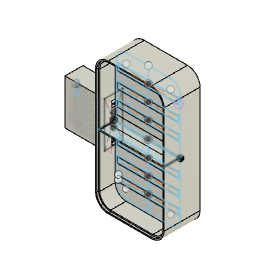
Sign (Autodesk Fusion 360 design; units mm, degrees)
Autodesk Fusion 360 part; units mm, degrees
note: some values were not read from the file. Chosen so that the rebuilt part matches the saved one: which face or edge a step refers to. Set by a fixed rule: which sketch regions a step uses.
sketch "body" plane through (0, 0, 0) normal (0, 1, 0) x (1, 0, 0)
  line L0 (36, 110) -> (-36, 110)
  line L1 (-57, 89) -> (-57, -89)
  line L2 (-36, -110) -> (36, -110)
  line L3 (57, -89) -> (57, 89)
  line L4 (57, 110) -> (-57, -110) construction
  line L5 (-57, 110) -> (57, -110) construction
  arc A0 (-57, -89) -> (-36, -110) centre (-36, -89) ccw
  arc A1 (36, -110) -> (57, -89) centre (36, -89) ccw
  arc A2 (57, 89) -> (36, 110) centre (36, 89) ccw
  arc A3 (-36, 110) -> (-57, 89) centre (-36, 89) ccw
  line L6 (-35.2, -106.2) -> (35.2, -106.2)
  line L7 (53.2, -88.2) -> (53.2, 88.2)
  line L8 (35.2, 106.2) -> (-35.2, 106.2)
  line L9 (-53.2, 88.2) -> (-53.2, -88.2)
  line L10 (-53.2, -106.2) -> (53.2, 106.2) construction
  line L11 (53.2, -106.2) -> (-53.2, 106.2) construction
  arc A4 (-53.2, -88.2) -> (-35.2, -106.2) centre (-35.2, -88.2) ccw
  arc A5 (35.2, -106.2) -> (53.2, -88.2) centre (35.2, -88.2) ccw
  arc A6 (-35.2, 106.2) -> (-53.2, 88.2) centre (-35.2, 88.2) ccw
  arc A7 (53.2, 88.2) -> (35.2, 106.2) centre (35.2, 88.2) ccw
  line L12 (35.2, 108.2) -> (-35.2, 108.2)
  line L13 (-55.2, 88.2) -> (-55.2, -88.2)
  line L14 (-35.2, -108.2) -> (35.2, -108.2)
  line L15 (55.2, -88.2) -> (55.2, 88.2)
  line L16 (55.2, 108.2) -> (-55.2, -108.2) construction
  line L17 (-55.2, 108.2) -> (55.2, -108.2) construction
  arc A8 (-55.2, -88.2) -> (-35.2, -108.2) centre (-35.2, -88.2) ccw
  arc A9 (35.2, -108.2) -> (55.2, -88.2) centre (35.2, -88.2) ccw
  arc A10 (55.2, 88.2) -> (35.2, 108.2) centre (35.2, 88.2) ccw
  arc A11 (-35.2, 108.2) -> (-55.2, 88.2) centre (-35.2, 88.2) ccw
  line L18 (-55, -1) -> (55, -1)
  line L19 (55, -1) -> (55, 1)
  line L20 (55, 1) -> (-55, 1)
  line L21 (-55, 1) -> (-55, -1)
  line L22 (-55, -1) -> (55, 1) construction
  line L23 (55, -1) -> (-55, 1) construction
  dimension "d1" = 220
  dimension "d2" = 114
  dimension "d3" = 21
  dimension "d4" = 21
  dimension "d5" = 21
  dimension "d6" = 21
  dimension "d10" = 106.4
  dimension "d11" = 212.4
  dimension "d12" = 18
  dimension "d13" = 18
  dimension "d14" = 18
  dimension "d15" = 18
  dimension "d48" = 110.4
  dimension "d49" = 216.4
  dimension "d50" = 20
  dimension "d51" = 20
  dimension "d52" = 20
  dimension "d53" = 20
  dimension "d65" = 2
  dimension "d76" = 110
  constraint perpendicular L0 L1
  constraint parallel L0 L2
  constraint parallel L1 L3
  constraint horizontal L0
  constraint coincident L4 origin
  constraint coincident L5 origin
  constraint coincident L4.end L2
  constraint coincident L4.end L1
  constraint tangent L2 A0
  constraint tangent L1 A0
  constraint coincident L5.end L2
  constraint coincident L5.end L3
  constraint tangent L2 A1
  constraint tangent L3 A1
  constraint coincident L4.start L3
  constraint coincident L4.start L0
  constraint tangent L3 A2
  constraint tangent L0 A2
  constraint coincident L5.start L1
  constraint coincident L5.start L0
  constraint tangent L1 A3
  constraint tangent L0 A3
  constraint perpendicular L6 L7
  constraint parallel L6 L8
  constraint parallel L7 L9
  constraint horizontal L6
  constraint coincident L10 origin
  constraint coincident L11 origin
  constraint coincident L10.start L6
  constraint coincident L10.start L9
  constraint tangent L6 A4
  constraint tangent L9 A4
  constraint coincident L11.start L6
  constraint coincident L11.start L7
  constraint tangent L6 A5
  constraint tangent L7 A5
  constraint coincident L11.end L9
  constraint coincident L11.end L8
  constraint tangent L9 A6
  constraint tangent L8 A6
  constraint coincident L10.end L7
  constraint coincident L10.end L8
  constraint tangent L7 A7
  constraint tangent L8 A7
  constraint perpendicular L12 L13
  constraint parallel L12 L14
  constraint parallel L13 L15
  constraint horizontal L12
  constraint coincident L16 origin
  constraint coincident L17 origin
  constraint coincident L16.end L14
  constraint coincident L16.end L13
  constraint tangent L14 A8
  constraint tangent L13 A8
  constraint coincident L17.end L14
  constraint coincident L17.end L15
  constraint tangent L14 A9
  constraint tangent L15 A9
  constraint coincident L16.start L12
  constraint coincident L16.start L15
  constraint tangent L12 A10
  constraint tangent L15 A10
  constraint coincident L17.start L13
  constraint coincident L17.start L12
  constraint tangent L13 A11
  constraint tangent L12 A11
  constraint perpendicular L18 L19
  constraint parallel L18 L20
  constraint parallel L19 L21
  constraint horizontal L18
  constraint coincident L22 origin
  constraint coincident L23 origin
  measures "d1" distance of L5.start L4.end
  measures "d2" distance of L4.end L5.end
  measures "d3" radius of A0
  measures "d4" radius of A1
  measures "d5" radius of A2
  measures "d6" radius of A3
  measures "d10" distance of L10.end L11.end
  measures "d11" distance of L11.start L10.end
  measures "d12" radius of A4
  measures "d13" radius of A5
  measures "d14" radius of A6
  measures "d15" radius of A7
  measures "d48" distance of L16.end L17.end
  measures "d49" distance of L17.start L16.end
  measures "d50" radius of A8
  measures "d51" radius of A9
  measures "d52" radius of A10
  measures "d53" radius of A11
  measures "d65" distance of L18.end L19.end
  measures "d76" distance of L18.start L18.end
  measures "d152" distance of origin
  measures "d220" distance of origin
  measures "d238" distance of origin
extrude "Extrude7" add sketch "body" along normal mid plane 60 contours L0 L1 L2 L3 A0 A1 A2 A3 makes body 1
extrude "Extrude8" add sketch "body" along normal mid plane 53.6 contours L9 L18 L20 L21 | L7 L18 L19 L20 | L12 L13 L14 L15 A8 A9 A10 A11 bodies 1
extrude "Extrude9" add sketch "body" along normal blind 25.8 from surface at 1 contours L7 L9 L18 L20 bodies 1
extrude "Extrude10" cut sketch "body" against normal blind 30 from surface at -1 contours L9 L18 L20 L21 | L7 L9 L18 L20 | L7 L18 L19 L20 bodies 1
extrude "Extrude1" add sketch "body" against normal blind 25.8 from surface at -1 separate body contours L9 L18 L20 L21 | L7 L9 L18 L20 | L7 L18 L19 L20 makes body 2 in component "led divider"
sketch "Ausschnitt kabel" plane through (-53.2, 0, 0) normal (1, 0, 0) x (0, 1, 0)
  line L0 (-26.8, 1) -> (-1, 1)
  line L1 (-1, 1) -> (-1, -1)
  line L2 (-1, -1) -> (-26.8, -1)
  line L3 (-26.8, -1) -> (-26.8, -88.2)
  line L4 (-26.8, -88.2) -> (26.8, -88.2)
  line L5 (26.8, -88.2) -> (26.8, -1)
  line L6 (26.8, -1) -> (1, -1)
  line L7 (1, -1) -> (1, 1)
  line L8 (1, 1) -> (26.8, 1)
  line L9 (26.8, 1) -> (26.8, 88.2)
  line L10 (26.8, 88.2) -> (-26.8, 88.2)
  line L11 (-7, 32.25) -> (7, 32.25)
  line L12 (7, 32.25) -> (7, -32.25)
  line L13 (7, -32.25) -> (-7, -32.25)
  line L14 (-7, -32.25) -> (-7, 32.25)
  line L15 (-7, 32.25) -> (7, -32.25) construction
  line L16 (7, 32.25) -> (-7, -32.25) construction
  line L17 (-7, 22.25) -> (7, 22.25)
  line L18 (7, 22.25) -> (7, -22.25)
  line L19 (7, -22.25) -> (-7, -22.25)
  line L20 (-7, -22.25) -> (-7, 22.25)
  line L21 (-7, 22.25) -> (7, -22.25) construction
  line L22 (7, 22.25) -> (-7, -22.25) construction
  line L23 (-26.8, 88.2) -> (-26.8, 1)
  dimension "d86" = 64.5
  dimension "d152" = 44.5
  dimension "d153" = 14
  constraint perpendicular L11 L12
  constraint parallel L11 L13
  constraint parallel L12 L14
  constraint horizontal L11
  constraint coincident L15 origin
  constraint coincident L16 origin
  constraint perpendicular L17 L18
  constraint parallel L17 L19
  constraint parallel L18 L20
  constraint horizontal L17
  constraint coincident L14 L17.start
  constraint coincident L21 origin
  constraint coincident L22 origin
  measures "d86" distance of L11.start L13.end
  measures "d152" distance of L17.start L19.end
  measures "d153" distance of L17.start L17.end
extrude "Extrude11" cut sketch "Ausschnitt kabel" against normal blind 19 contours L11 L12 L14 L17 | L12 L13 L14 L19 bodies 1
extrude "Extrude1'" add sketch "body" along normal mid plane 2 separate body contours L6 L7 L9 A4 A5 L18 | L7 L9 L18 L20 | L7 L8 L9 A6 A7 L20 makes body 3 in component "LED plate"
extrude "Extrude1''" add sketch "body" along normal blind 3 separate body contours L6 L7 L9 A4 A5 L18 | L9 L18 L20 L21 | L7 L9 L18 L20 | L7 L18 L19 L20 | L7 L8 L9 A6 A7 L20 | L12 L13 L14 L15 A8 A9 A10 A11 makes body 4 in component "glass"
sketch "vorderseite" plane through (0, -1, 0) normal (0, -1, 0) x (1, 0, 0) in component "LED plate"
  arc A0 (35.2, -106.2) -> (53.2, -88.2) centre (35.2, -88.2) ccw
  line L0 (53.2, -88.2) -> (53.2, 88.2)
  arc A1 (53.2, 88.2) -> (35.2, 106.2) centre (35.2, 88.2) ccw
  line L1 (35.2, 106.2) -> (-35.2, 106.2)
  arc A2 (-35.2, 106.2) -> (-53.2, 88.2) centre (-35.2, 88.2) ccw
  line L2 (-53.2, 88.2) -> (-53.2, -88.2)
  arc A3 (-53.2, -88.2) -> (-35.2, -106.2) centre (-35.2, -88.2) ccw
  line L3 (-35.2, -106.2) -> (35.2, -106.2)
  line L4 (-53, 1) -> (53, 1)
  line L5 (53, 1) -> (53, -1)
  line L6 (53, -1) -> (-53, -1)
  line L7 (-53, -1) -> (-53, 1)
  line L8 (-53, 1) -> (53, -1) construction
  line L9 (53, 1) -> (-53, -1) construction
  line L10 (0, -1) -> (0, -106.2)
  line L11 (0, -106.2) -> (0, -79.95)
  line L12 (0, -79.95) -> (0, -53.7)
  line L13 (0, -53.7) -> (0, -27.45)
  line L14 (0, -27.45) -> (0, -1.2)
  line L15 (-49.993, -74.9491) -> (49.993, -74.9491)
  line L16 (49.993, -74.9491) -> (49.993, -84.9509)
  line L17 (49.993, -84.9509) -> (-49.993, -84.9509)
  line L18 (-49.993, -84.9509) -> (-49.993, -74.9491)
  line L19 (-49.993, -74.9491) -> (49.993, -84.9509) construction
  line L20 (49.993, -74.9491) -> (-49.993, -84.9509) construction
  line L21 (-49.9993, -48.693) -> (49.9993, -48.693)
  line L22 (49.9993, -48.693) -> (49.9993, -58.707)
  line L23 (49.9993, -58.707) -> (-49.9993, -58.707)
  line L24 (-49.9993, -58.707) -> (-49.9993, -48.693)
  line L25 (-49.9993, -48.693) -> (49.9993, -58.707) construction
  line L26 (49.9993, -48.693) -> (-49.9993, -58.707) construction
  line L27 (-49.9996, -22.4465) -> (49.9996, -22.4465)
  line L28 (49.9996, -22.4465) -> (49.9996, -32.4535)
  line L29 (49.9996, -32.4535) -> (-49.9996, -32.4535)
  line L30 (-49.9996, -32.4535) -> (-49.9996, -22.4465)
  line L31 (-49.9996, -22.4465) -> (49.9996, -32.4535) construction
  line L32 (49.9996, -22.4465) -> (-49.9996, -32.4535) construction
  line L33 (0, 1) -> (0, 27.25)
  line L34 (0, 27.25) -> (0, 53.5)
  line L35 (0, 53.5) -> (0, 79.75)
  line L36 (0, 79.75) -> (0, 106)
  line L37 (-49.954, 74.7499) -> (49.954, 74.7499)
  line L38 (49.954, 74.7499) -> (49.954, 84.7501)
  line L39 (49.954, 84.7501) -> (-49.954, 84.7501)
  line L40 (-49.954, 84.7501) -> (-49.954, 74.7499)
  line L41 (-49.954, 74.7499) -> (49.954, 84.7501) construction
  line L42 (49.954, 74.7499) -> (-49.954, 84.7501) construction
  line L43 (-50, 58.5) -> (50, 58.5)
  line L44 (50, 58.5) -> (50, 48.5)
  line L45 (50, 48.5) -> (-50, 48.5)
  line L46 (-50, 48.5) -> (-50, 58.5)
  line L47 (-50, 58.5) -> (50, 48.5) construction
  line L48 (50, 58.5) -> (-50, 48.5) construction
  line L49 (-50, 32.25) -> (50, 32.25)
  line L50 (50, 32.25) -> (50, 22.25)
  line L51 (50, 22.25) -> (-50, 22.25)
  line L52 (-50, 22.25) -> (-50, 32.25)
  line L53 (-50, 32.25) -> (50, 22.25) construction
  line L54 (50, 32.25) -> (-50, 22.25) construction
  line L55 (50, -76.25) -> (50, -83.25)
  line L56 (53.2, 84.75) -> (53.2, 74.75)
  line L57 (49.954, 79.75) -> (53.2, 79.75)
  line L58 (53.2, 79.75) -> (52.2, 79.75)
  line L59 (52.2, 79.75) -> (52.2042, 84.7482)
  line L60 (52.2, 79.75) -> (52.1874, 74.7499)
  line L61 (49.954, 84.7501) -> (52.2042, 84.7482)
  line L62 (49.954, 74.7499) -> (52.1874, 74.7499)
  line L63 (52.0711, 75.7486) -> (52.0778, 83.7487)
  arc A4 (52.0778, 83.7487) -> (50.0787, 83.7504) centre (51.0782, 83.7496) ccw
  line L64 (50.0787, 83.7504) -> (50.072, 75.7503)
  arc A5 (50.072, 75.7503) -> (52.0711, 75.7486) centre (51.0715, 75.7495) ccw
  line L65 (51.0707, 74.7499) -> (51.0791, 84.7491) construction
  line L66 (49.993, -74.9491) -> (51.993, -74.9491)
  line L67 (51.993, -74.9491) -> (51.993, -84.9509)
  line L68 (49.993, -84.9509) -> (51.993, -84.9509)
  line L69 (51.9959, -83.948) -> (51.9959, -75.952)
  arc A6 (51.9959, -75.952) -> (49.9901, -75.952) centre (50.993, -75.952) ccw
  line L70 (49.9901, -75.952) -> (49.9901, -83.948)
  arc A7 (49.9901, -83.948) -> (51.9959, -83.948) centre (50.993, -83.948) ccw
  line L71 (50.993, -84.9509) -> (50.993, -74.9491) construction
  line L72 (-49.5, 84.25) -> (49.5, 84.25)
  line L73 (49.5, 84.25) -> (49.5, 75.25)
  line L74 (49.5, 75.25) -> (-49.5, 75.25)
  line L75 (-49.5, 75.25) -> (-49.5, 84.25)
  line L76 (-49.5, 84.25) -> (49.5, 75.25) construction
  line L77 (49.5, 84.25) -> (-49.5, 75.25) construction
  line L78 (-49.5, 58) -> (49.5, 58)
  line L79 (49.5, 58) -> (49.5, 49)
  line L80 (49.5, 49) -> (-49.5, 49)
  line L81 (-49.5, 49) -> (-49.5, 58)
  line L82 (-49.5, 58) -> (49.5, 49) construction
  line L83 (49.5, 58) -> (-49.5, 49) construction
  line L84 (-49.5, 31.75) -> (49.5, 31.75)
  line L85 (49.5, 31.75) -> (49.5, 22.75)
  line L86 (49.5, 22.75) -> (-49.5, 22.75)
  line L87 (-49.5, 22.75) -> (-49.5, 31.75)
  line L88 (-49.5, 31.75) -> (49.5, 22.75) construction
  line L89 (49.5, 31.75) -> (-49.5, 22.75) construction
  line L90 (-49.4997, -22.9468) -> (49.4997, -22.9468)
  line L91 (49.4997, -22.9468) -> (49.4997, -31.9532)
  line L92 (49.4997, -31.9532) -> (-49.4997, -31.9532)
  line L93 (-49.4997, -31.9532) -> (-49.4997, -22.9468)
  line L94 (-49.4997, -22.9468) -> (49.4997, -31.9532) construction
  line L95 (49.4997, -22.9468) -> (-49.4997, -31.9532) construction
  line L96 (-49.4994, -49.1936) -> (49.4994, -49.1936)
  line L97 (49.4994, -49.1936) -> (49.4994, -58.2064)
  line L98 (49.4994, -58.2064) -> (-49.4994, -58.2064)
  line L99 (-49.4994, -58.2064) -> (-49.4994, -49.1936)
  line L100 (-49.4994, -49.1936) -> (49.4994, -58.2064) construction
  line L101 (49.4994, -49.1936) -> (-49.4994, -58.2064) construction
  line L102 (-49.5, -75.4499) -> (49.5, -75.4499)
  line L103 (49.5, -75.4499) -> (49.5, -84.4501)
  line L104 (49.5, -84.4501) -> (-49.5, -84.4501)
  line L105 (-49.5, -84.4501) -> (-49.5, -75.4499)
  line L106 (-49.5, -75.4499) -> (49.5, -84.4501) construction
  line L107 (49.5, -75.4499) -> (-49.5, -84.4501) construction
  line L108 (49.5, 84.25) -> (49.5, 84.7501)
  line L109 (49.5, 75.25) -> (49.5, 74.7499)
  line L110 (49.5, -75.4499) -> (49.5, -74.9491)
  line L111 (49.5, -84.4501) -> (49.5, -84.9509)
  point P0 (0, -27.45)
  point P1 (0, -53.7)
  point P2 (0, -79.95)
  point P3 (0, -79.95)
  point P4 (0, -53.7)
  point P5 (0, -27.45)
  point P6 (0, 79.75)
  point P7 (0, 53.5)
  point P8 (0, 27.25)
  point P9 (0, 79.75)
  point P10 (0, 53.5)
  point P11 (0, 27.25)
  point P12 (0, 79.75)
  point P13 (0, 53.5)
  point P14 (0, 27.25)
  point P15 (0, -27.45)
  point P16 (0, -53.7)
  point P17 (0, -79.95)
  dimension "d91" = 2
  dimension "d92" = 105
  dimension "d93" = 26.25
  dimension "d94" = 26.25
  dimension "d95" = 26.25
  dimension "d96" = 26.25
  dimension "d103" = 26.25
  dimension "d104" = 26.25
  dimension "d105" = 26.25
  dimension "d106" = 26.25
  dimension "d113" = 1
  dimension "d114" = 2
  constraint perpendicular L4 L5
  constraint parallel L4 L6
  constraint parallel L5 L7
  constraint horizontal L4
  constraint coincident L8 origin
  constraint coincident L9 origin
  constraint midpoint L6 L10.start
  constraint midpoint L3 L10.end
  constraint perpendicular L3 L11
  constraint parallel L10 L12
  constraint parallel L10 L13
  constraint parallel L10 L14
  constraint coincident P15 P5
  constraint coincident P16 P4
  constraint coincident P17 P3
  constraint perpendicular L15 L16
  constraint parallel L15 L17
  constraint parallel L16 L18
  constraint horizontal L15
  constraint coincident L19 P17
  constraint coincident L20 P17
  constraint perpendicular L21 L22
  constraint parallel L21 L23
  constraint parallel L22 L24
  constraint horizontal L21
  constraint coincident L25 P16
  constraint coincident L26 P16
  constraint perpendicular L27 L28
  constraint parallel L27 L29
  constraint parallel L28 L30
  constraint horizontal L27
  constraint coincident L31 P15
  constraint coincident L32 P15
  constraint midpoint L4 L33.start
  constraint perpendicular L4 L33
  constraint parallel L33 L34
  constraint parallel L34 L35
  constraint parallel L35 L36
  constraint coincident P12 P9
  constraint coincident P13 P10
  constraint coincident P14 P11
  constraint perpendicular L37 L38
  constraint parallel L37 L39
  constraint parallel L38 L40
  constraint horizontal L37
  constraint coincident L41 P12
  constraint coincident L42 P12
  constraint perpendicular L43 L44
  constraint parallel L43 L45
  constraint parallel L44 L46
  constraint horizontal L43
  constraint coincident L47 P13
  constraint coincident L48 P13
  constraint perpendicular L49 L50
  constraint parallel L49 L51
  constraint parallel L50 L52
  constraint horizontal L49
  constraint coincident L53 P14
  constraint coincident L54 P14
  constraint coincident L0 L56.start
  constraint coincident L0 L56.end
  constraint midpoint L38 L57.start
  constraint midpoint L56 L57.end
  constraint perpendicular L56 L57
  constraint perpendicular L56 L58
  constraint perpendicular L59 L61
  constraint perpendicular L38 L62
  constraint tangent L63 A4
  constraint tangent A4 L64
  constraint parallel L63 L64
  constraint tangent L64 A5
  constraint tangent L63 A5
  constraint midpoint A5 L65.start
  constraint midpoint A4 L65.end
  constraint midpoint L61 L65.end
  constraint perpendicular L61 L65
  constraint midpoint L62 L65.start
  constraint perpendicular L16 L66
  constraint perpendicular L66 L67
  constraint perpendicular L67 L68
  constraint tangent L69 A6
  constraint tangent A6 L70
  constraint parallel L69 L70
  constraint tangent L70 A7
  constraint tangent L69 A7
  constraint midpoint A7 L71.start
  constraint midpoint A6 L71.end
  constraint midpoint L66 L71.end
  constraint perpendicular L66 L71
  constraint midpoint L68 L71.start
  constraint perpendicular L72 L73
  constraint parallel L72 L74
  constraint parallel L73 L75
  constraint horizontal L72
  constraint coincident L76 P12
  constraint coincident L77 P12
  constraint perpendicular L78 L79
  constraint parallel L78 L80
  constraint parallel L79 L81
  constraint horizontal L78
  constraint coincident L82 P13
  constraint coincident L83 P13
  constraint perpendicular L84 L85
  constraint parallel L84 L86
  constraint parallel L85 L87
  constraint horizontal L84
  constraint coincident L88 P14
  constraint coincident L89 P14
  constraint perpendicular L90 L91
  constraint parallel L90 L92
  constraint parallel L91 L93
  constraint horizontal L90
  constraint coincident L94 P15
  constraint coincident L95 P15
  constraint perpendicular L96 L97
  constraint parallel L96 L98
  constraint parallel L97 L99
  constraint horizontal L96
  constraint coincident L100 P16
  constraint coincident L101 P16
  constraint perpendicular L102 L103
  constraint parallel L102 L104
  constraint parallel L103 L105
  constraint horizontal L102
  constraint coincident L106 P17
  constraint coincident L107 P17
  constraint coincident L39 L108.end
  constraint perpendicular L39 L108
  constraint coincident L37 L109.end
  constraint perpendicular L37 L109
  constraint coincident L15 L110.end
  constraint perpendicular L15 L110
  constraint coincident L17 L111.end
  constraint perpendicular L17 L111
  measures "d91" distance of L4.end L5.end
  measures "d93" distance of L10.end P17
  measures "d94" distance of P17 P16
  measures "d95" distance of P16 P15
  measures "d96" distance of P15 L14.end
  measures "d103" distance of L33.start P14
  measures "d104" distance of P14 P13
  measures "d105" distance of P13 P12
  measures "d106" distance of P12 L36.end
  measures "d113" distance of L57.end L58.end
  measures "d114" distance of L15.end L66.end
extrude "Extrude2" cut sketch "vorderseite" against normal blind 10 contours L57 L63 L64 A5 | L57 L63 A4 L64 bodies 3 in component "LED plate"
extrude "Extrude3" cut sketch "vorderseite" against normal blind 0.2 contours L10 L11 L12 L15 L17 L18 L102 L104 L105 | L10 L11 L17 L104 L111 | L15 L16 L17 A6 L70 A7 L103 L110 L111 | L10 L12 L15 L102 L110 | L16 A6 L70 A7 | L10 L12 L13 L21 L23 L24 L96 L98 L99 | L10 L12 L13 L21 L22 L23 L96 L97 L98 | L37 L38 L39 L73 L108 L109 | L36 L39 L72 L108 | L35 L37 L74 L109 | L35 L36 L37 L39 L40 L72 L74 L75 | L34 L35 L43 L44 L45 L78 L79 L80 | L34 L35 L43 L45 L46 L78 L80 L81 | L10 L13 L14 L27 L29 L30 L90 L92 L93 | L10 L13 L14 L27 L28 L29 L90 L91 L92 | L33 L34 L49 L50 L51 L84 L85 L86 | L33 L34 L49 L51 L52 L84 L86 L87 bodies 3 in component "LED plate"
extrude "Extrude4" add sketch "vorderseite" against normal blind 0.2 contours L37 L38 L39 L73 L108 L109 bodies 3 in component "LED plate"
extrude "Extrude5" add sketch "vorderseite" against normal blind 0.2 contours L15 L16 L17 L55 L70 L103 L110 L111 bodies 3 in component "LED plate"
sketch "Sketch2" plane through (0, 1, 0) normal (0, 1, 0) x (-1, 0, 0) in component "LED plate"
  line L0 (-52.0711, 75.7486) -> (-52.0778, 83.7487)
  arc A0 (-50.0787, 83.7504) -> (-52.0778, 83.7487) centre (-51.0782, 83.7496) ccw
  line L1 (-50.0787, 83.7504) -> (-50.072, 75.7503)
  arc A1 (-52.0711, 75.7486) -> (-50.072, 75.7503) centre (-51.0715, 75.7495) ccw
  arc A2 (-53.2, -88.2) -> (-35.2, -106.2) centre (-35.2, -88.2) ccw
  line L2 (-35.2, -106.2) -> (35.2, -106.2)
  arc A3 (35.2, -106.2) -> (53.2, -88.2) centre (35.2, -88.2) ccw
  line L3 (53.2, -88.2) -> (53.2, 88.2)
  arc A4 (53.2, 88.2) -> (35.2, 106.2) centre (35.2, 88.2) ccw
  line L4 (35.2, 106.2) -> (-35.2, 106.2)
  arc A5 (-35.2, 106.2) -> (-53.2, 88.2) centre (-35.2, 88.2) ccw
  line L5 (-53.2, 88.2) -> (-53.2, -88.2)
  line L6 (50, -74.75) -> (-50, -84.75) construction
  line L7 (50, -84.75) -> (-50, -84.75)
  line L8 (-50, -74.75) -> (50, -84.75) construction
  line L9 (49.5, -75.25) -> (-49.5, -84.25) construction
  line L10 (49.5, -84.25) -> (-49.5, -84.25)
  line L11 (-49.5, -75.25) -> (49.5, -84.25) construction
  line L12 (-50, -84.75) -> (-50, -74.75)
  line L13 (-49.5, -75.25) -> (49.5, -75.25)
  line L14 (49.5, -49) -> (-49.5, -58) construction
  line L15 (-49.5, -49) -> (49.5, -49)
  line L16 (50, -48.5) -> (-50, -58.5) construction
  line L17 (50, -58.5) -> (-50, -58.5)
  line L18 (49.5, -84.25) -> (49.5, -84.75)
  line L19 (49.5, -58) -> (-49.5, -58)
  line L20 (49.5, 84.25) -> (49.5, 84.75)
  line L21 (50, -76.25) -> (50, -83.25)
  line L22 (50, -74.75) -> (50, -84.75)
  line L23 (49.5, -75.25) -> (49.5, -84.25)
  arc A6 (-53, -90) -> (-37, -106) centre (-37, -90) ccw
  line L24 (-50, -48.5) -> (50, -58.5) construction
  line L25 (-50, -48.5) -> (50, -48.5)
  line L26 (-50, -74.75) -> (50, -74.75)
  line L27 (-49.5, -22.75) -> (49.5, -22.75)
  line L28 (49.5, -49) -> (49.5, -58)
  line L29 (50, -75.75) -> (50, -83.75)
  line L30 (-37, -106) -> (37, -106)
  line L31 (50, -48.5) -> (50, -58.5)
  line L32 (49.5, -75.25) -> (49.5, -74.75)
  line L33 (-49.5, -49) -> (49.5, -58) construction
  line L34 (-49.5, -22.75) -> (49.5, -31.75) construction
  line L35 (49.5, -22.75) -> (49.5, -31.75)
  arc A7 (37, -106) -> (53, -90) centre (37, -90) ccw
  line L36 (-49.5, -84.25) -> (-49.5, -75.25)
  line L37 (0, -79.75) -> (0, -53.5)
  line L38 (0, -106) -> (0, -79.75)
  line L39 (-49.5, -58) -> (-49.5, -49)
  line L40 (-50, -58.5) -> (-50, -48.5)
  line L41 (0, 53.5) -> (0, 79.75)
  line L42 (-49.5, 49) -> (-49.5, 58)
  line L43 (0, 79.75) -> (0, 106)
  line L44 (49.5, 75.25) -> (49.5, 74.75)
  line L45 (0, -1) -> (0, -106)
  line L46 (53, 84.75) -> (53, 74.75)
  line L47 (50, -22.25) -> (50, -32.25)
  arc A8 (53, 90) -> (37, 106) centre (37, 90) ccw
  line L48 (-50, -22.25) -> (50, -22.25)
  line L49 (0, -27.25) -> (0, -1)
  line L50 (53, 1) -> (-53, -1) construction
  line L51 (-53, 1) -> (53, -1) construction
  line L52 (-53, -1) -> (-53, 1)
  line L53 (53, 1) -> (53, -1)
  arc A9 (-37, 106) -> (-53, 90) centre (-37, 90) ccw
  line L54 (-49.5, -31.75) -> (-49.5, -22.75)
  line L55 (49.5, 22.75) -> (-49.5, 22.75)
  line L56 (0, 1) -> (0, 27.25)
  line L57 (-50, -32.25) -> (-50, -22.25)
  line L58 (50, -32.25) -> (-50, -32.25)
  line L59 (-53, 1) -> (53, 1)
  line L60 (49.5, -22.75) -> (-49.5, -31.75) construction
  line L61 (49.5, -31.75) -> (-49.5, -31.75)
  line L62 (-50, -22.25) -> (50, -32.25) construction
  line L63 (53, -1) -> (-53, -1)
  line L64 (37, 106) -> (-37, 106)
  line L65 (-53, 90) -> (-53, -90)
  line L66 (53, -90) -> (53, 90)
  line L67 (-50, 48.5) -> (-50, 58.5)
  line L68 (50, 22.25) -> (-50, 22.25)
  line L69 (50, -22.25) -> (-50, -32.25) construction
  line L70 (-50, 84.75) -> (-50, 74.75)
  line L71 (-49.5, 75.25) -> (-49.5, 84.25)
  line L72 (0, -53.5) -> (0, -27.25)
  line L73 (49.5, 58) -> (49.5, 49)
  line L74 (49.5, 84.25) -> (49.5, 75.25)
  line L75 (50, 58.5) -> (50, 48.5)
  line L76 (-49.5, 31.75) -> (49.5, 31.75)
  line L77 (-49.5, 58) -> (49.5, 49) construction
  line L78 (-49.5, 58) -> (49.5, 58)
  line L79 (-49.5, 84.25) -> (49.5, 75.25) construction
  line L80 (50, 48.5) -> (-50, 48.5)
  line L81 (-50, 74.75) -> (50, 74.75)
  line L82 (49.5, 58) -> (-49.5, 49) construction
  line L83 (50, 74.75) -> (-50, 84.75) construction
  line L84 (-50, 74.75) -> (50, 84.75) construction
  line L85 (50, 32.25) -> (50, 22.25)
  line L86 (49.5, 49) -> (-49.5, 49)
  line L87 (49.5, 31.75) -> (49.5, 22.75)
  line L88 (-49.5, 84.25) -> (49.5, 84.25)
  line L89 (-49.5, 22.75) -> (-49.5, 31.75)
  line L90 (50, 58.5) -> (-50, 48.5) construction
  line L91 (-50, 58.5) -> (50, 48.5) construction
  line L92 (-50, 58.5) -> (50, 58.5)
  line L93 (-50, 32.25) -> (50, 22.25) construction
  line L94 (50, 84.75) -> (-50, 84.75)
  line L95 (50, 32.25) -> (-50, 22.25) construction
  line L96 (49.5, 84.25) -> (-49.5, 75.25) construction
  line L97 (49.5, 75.25) -> (-49.5, 75.25)
  line L98 (-50, 22.25) -> (-50, 32.25)
  line L99 (-49.5, 31.75) -> (49.5, 22.75) construction
  line L100 (-50, 32.25) -> (50, 32.25)
  line L101 (0, 27.25) -> (0, 53.5)
  line L102 (49.5, 31.75) -> (-49.5, 22.75) construction
  line L103 (50, 74.75) -> (50, 84.75)
  line L104 (-49.5, 84.25) -> (-49.5, 84.75)
  line L105 (-49.5, 75.25) -> (-49.5, 74.75)
  line L106 (-49.5, -75.25) -> (-49.5, -74.75)
  line L107 (-49.5, -84.25) -> (-49.5, -84.75)
  point P0 (0, 79.75)
  point P1 (0, -53.5)
  point P2 (0, 79.75)
  point P3 (0, -27.25)
  point P4 (0, 53.5)
  point P5 (0, -27.25)
  point P6 (0, 27.25)
  point P7 (0, -53.5)
  point P8 (0, -79.75)
  point P9 (0, -79.75)
  point P10 (0, -27.25)
  point P11 (0, 27.25)
  point P12 (0, 53.5)
  point P13 (0, 27.25)
  point P14 (0, 79.75)
  point P15 (0, 53.5)
  point P16 (0, -53.5)
  point P17 (0, -79.75)
  dimension "d135" = 2
  dimension "d136" = 26.25
  dimension "d137" = 26.25
  dimension "d138" = 26.25
  dimension "d139" = 26.25
  dimension "d140" = 26.25
  dimension "d141" = 26.25
  dimension "d142" = 26.25
  dimension "d143" = 26.25
  constraint perpendicular L53 L59
  constraint parallel L59 L63
  constraint parallel L52 L53
  constraint horizontal L59
  constraint coincident origin L51
  constraint coincident origin L50
  constraint midpoint L45.start L63
  constraint midpoint L38.start L30
  constraint perpendicular L30 L38
  constraint parallel L37 L45
  constraint parallel L45 L72
  constraint parallel L45 L49
  constraint coincident P10 P5
  constraint coincident P16 P7
  constraint coincident P17 P9
  constraint perpendicular L22 L26
  constraint parallel L7 L26
  constraint parallel L12 L22
  constraint horizontal L26
  constraint coincident P17 L8
  constraint coincident P17 L6
  constraint perpendicular L25 L31
  constraint parallel L17 L25
  constraint parallel L31 L40
  constraint horizontal L25
  constraint coincident P16 L24
  constraint coincident P16 L16
  constraint perpendicular L47 L48
  constraint parallel L48 L58
  constraint parallel L47 L57
  constraint horizontal L48
  constraint coincident P10 L62
  constraint coincident P10 L69
  constraint midpoint L56.start L59
  constraint perpendicular L56 L59
  constraint parallel L56 L101
  constraint parallel L41 L101
  constraint parallel L41 L43
  constraint coincident P14 P2
  constraint coincident P15 P12
  constraint coincident P13 P11
  constraint parallel L81 L94
  constraint horizontal L81
  constraint coincident P14 L84
  constraint coincident P14 L83
  constraint perpendicular L75 L92
  constraint parallel L80 L92
  constraint parallel L67 L75
  constraint horizontal L92
  constraint coincident P15 L91
  constraint coincident P15 L90
  constraint perpendicular L85 L100
  constraint parallel L68 L100
  constraint parallel L85 L98
  constraint horizontal L100
  constraint coincident P13 L93
  constraint coincident P13 L95
  constraint coincident L46.start L66
  constraint coincident L46.end L66
  constraint perpendicular L74 L88
  constraint parallel L88 L97
  constraint parallel L71 L74
  constraint horizontal L88
  constraint coincident P14 L79
  constraint coincident P14 L96
  constraint perpendicular L73 L78
  constraint parallel L78 L86
  constraint parallel L42 L73
  constraint horizontal L78
  constraint coincident P15 L77
  constraint coincident P15 L82
  constraint perpendicular L76 L87
  constraint parallel L55 L76
  constraint parallel L87 L89
  constraint horizontal L76
  constraint coincident P13 L99
  constraint coincident P13 L102
  constraint perpendicular L27 L35
  constraint parallel L27 L61
  constraint parallel L35 L54
  constraint horizontal L27
  constraint coincident P10 L34
  constraint coincident P10 L60
  constraint perpendicular L15 L28
  constraint parallel L15 L19
  constraint parallel L28 L39
  constraint horizontal L15
  constraint coincident P16 L33
  constraint coincident P16 L14
  constraint perpendicular L13 L23
  constraint parallel L10 L13
  constraint parallel L23 L36
  constraint horizontal L13
  constraint coincident P17 L11
  constraint coincident P17 L9
  constraint coincident L20.end L94
  constraint perpendicular L20 L94
  constraint coincident L44.end L81
  constraint perpendicular L44 L81
  constraint coincident L32.end L26
  constraint perpendicular L26 L32
  constraint coincident L18.end L7
  constraint perpendicular L7 L18
  constraint perpendicular L94 L103
  constraint coincident L94 L104.end
  constraint perpendicular L94 L104
  constraint coincident L81 L105.end
  constraint perpendicular L81 L105
  constraint coincident L26 L106.end
  constraint perpendicular L26 L106
  constraint coincident L7 L107.end
  constraint perpendicular L7 L107
  measures "d135" distance of L50.start L51.end
  measures "d136" distance of L38.start P17
  measures "d137" distance of P16 P17
  measures "d138" distance of P10 P16
  measures "d139" distance of P10 L45.start
  measures "d140" distance of L56.start P13
  measures "d141" distance of P15 P13
  measures "d142" distance of P14 P15
  measures "d143" distance of P14 L43.end
extrude "Extrude7'" add sketch "Sketch2" against normal blind 0.2 contours L7 L12 L26 L36 L106 L107 | L70 L71 L81 L94 L104 L105 bodies 3 in component "LED plate"
extrude "Extrude6" cut sketch "Sketch2" against normal blind 0.2 contours L7 L10 L18 L38 L45 | L7 L10 L38 L45 L107 | L27 L35 L45 L47 L48 L49 L58 L61 L72 | L27 L45 L48 L49 L54 L57 L58 L61 L72 | L7 L18 L21 L22 L23 L26 L29 L32 | L7 L12 L26 L36 L106 L107 | L55 L56 L68 L76 L89 L98 L100 L101 | L55 L56 L68 L76 L85 L87 L100 L101 | L20 L43 L88 L94 | L43 L88 L94 L104 | L20 L44 L74 L81 L94 L103 | L70 L71 L81 L94 L104 L105 | L13 L26 L32 L37 L45 | L13 L26 L37 L45 L106 | L15 L17 L19 L25 L37 L39 L40 L45 L72 | L15 L17 L19 L25 L28 L31 L37 L45 L72 | L41 L44 L81 L97 | L41 L81 L97 L105 | L41 L73 L75 L78 L80 L86 L92 L101 | L41 L42 L67 L78 L80 L86 L92 L101 bodies 3 in component "LED plate"
extrude "Extrude8'" add sketch "Sketch2" against normal blind 0.2 contours L7 L12 L26 L36 L106 L107 | L70 L71 L81 L94 L104 L105 bodies 3 in component "LED plate"
copy_body "Body->Comp2" bodies 1 removing the originals makes body 5 in component "case"
sketch "Sketch1" plane through (-57, 0, 0) normal (-1, 0, 0) x (0, -1, 0) in component "case"
  line L0 (7, 22.25) -> (-7, 22.25)
  line L1 (-7, 22.25) -> (-7, 32.25)
  line L2 (-7, 32.25) -> (7, 32.25)
  line L3 (7, 32.25) -> (7, 22.25)
  line L4 (-7, -22.25) -> (7, -22.25)
  line L5 (7, -22.25) -> (7, -32.25)
  line L6 (7, -32.25) -> (-7, -32.25)
  line L7 (-7, -32.25) -> (-7, -22.25)
  line L8 (30, 89) -> (-30, 89)
  line L9 (-30, 89) -> (-30, -89)
  line L10 (-30, -89) -> (30, -89)
  line L11 (30, -89) -> (30, 89)
  line L12 (0, 0) -> (0, 22.25)
  circle A0 centre (0, 11.125) radius 3.1
  line L13 (0, 0) -> (0, -22.25)
  circle A1 centre (0, -11.125) radius 3.1
  dimension "d154" = 6.2
  dimension "d155" = 6.2
  constraint coincident L12.start L13.start
  constraint midpoint L0 L12.end
  constraint midpoint L12 A0.centre
  constraint midpoint L4 L13.end
  constraint midpoint L13 A1.centre
  measures "d154" diameter of A0
  measures "d155" diameter of A1
extrude "Extrude1'''" cut sketch "Sketch1" against normal blind 2 contours L12 A0 | L12 A0 | L13 A1 | L13 A1 bodies 5 in component "case"
extrude "Extrude2'" cut 2 faces at (-54.4, -9.6, 1) (53.8, -9.6, 1) along direction (0, 0, 1) blind 0.2 on bodies 5 bodies 5 in component "case"
extrude "Extrude3'" cut 2 faces at (-53.8, -9.6, -1) (54.4, -9.6, -1) along direction (0, 0, -1) blind 0.2 on bodies 5 bodies 5 in component "case"
sketch "Sketch1 (2)" plane through (0, 0, 1) normal (0, 0, 1) x (-1, 0, 0) in component "led divider"
  line L0 (-55, 1) -> (55, 1)
  line L1 (55, 1) -> (55, 26.8)
  line L2 (55, 26.8) -> (-55, 26.8)
  line L3 (-55, 26.8) -> (-55, 1)
  line L4 (53, 3) -> (-53, 3)
  line L5 (-53, 3) -> (-53, 1)
  line L6 (-53, 1) -> (53, 1)
  line L7 (53, 1) -> (53, 3)
  line L8 (53, 3) -> (-53, 1) construction
  line L9 (-53, 3) -> (53, 1) construction
  line L10 (-55, 1) -> (-53, 1)
  line L11 (-53, 1) -> (-53, 26.8)
  line L12 (-53, 26.8) -> (-55, 26.8)
  line L13 (-55, 26.8) -> (-55, 1)
  line L14 (55, 1) -> (53, 1)
  line L15 (53, 1) -> (53, 26.8)
  line L16 (53, 26.8) -> (55, 26.8)
  line L17 (55, 26.8) -> (55, 1)
  point P0 (0, 2)
  dimension "d169" = 2
  dimension "d181" = 2
  dimension "d182" = 2
  constraint perpendicular L4 L5
  constraint parallel L4 L6
  constraint parallel L5 L7
  constraint horizontal L4
  constraint coincident L8 P0
  constraint coincident L9 P0
  constraint horizontal L10
  constraint vertical L11
  constraint horizontal L12
  constraint vertical L13
  constraint coincident L0.start L3.end
  constraint horizontal L14
  constraint vertical L15
  constraint horizontal L16
  constraint vertical L17
  constraint coincident L0.end L1.start
  measures "d169" distance of L4.start L6.end
  measures "d181" distance of L0.start L5.end
  measures "d182" distance of L0.end L6.end
extrude "Extrude2''" add sketch "Sketch1 (2)" along normal blind 10 contours L0 L4 L5 L6 L7 L11 L15 bodies 2 in component "led divider"
extrude "Extrude3''" add sketch "Sketch1 (2)" against normal blind 12 contours L0 L4 L5 L6 L7 L11 L15 bodies 2 in component "led divider"
extrude "Extrude4'" cut 2 faces at (-17.6667, -3, 4.3333) (-17.6667, -3, -4.3333) along direction (0, 1, 0) blind 1.8 on bodies 2 bodies 2 in component "led divider"
extrude "Extrude5'" cut sketch "Sketch1 (2)" against normal blind 0.2 contours L0 L2 L3 L5 L10 L11 L12 L13 | L0 L1 L2 L7 L14 L15 L16 L17 bodies 2 in component "led divider"
extrude "Extrude6'" cut sketch "Sketch1 (2)" along normal blind 0.2 from surface at -2 contours L0 L2 L3 L5 L10 L11 L12 L13 | L0 L1 L2 L7 L14 L15 L16 L17 bodies 2 in component "led divider"
fillet "Fillet3" radius 10 2 edges at (0, -1.2, 1) (0, -1.2, -1) on bodies 2 in component "led divider"
fillet "Fillet5" radius 0.8 4 edges at (55, -13.9, 0.8) (55, -13.9, -0.8) (-55, -13.9, 0.8) (-55, -13.9, -0.8) on bodies 2 in component "led divider"
sketch "Sketch2 (2)" plane through (-57, 0, 0) normal (-1, 0, 0) x (0, -1, 0) in component "ESP Case"
  circle A0 centre (0, 11.125) radius 3.1
  circle A1 centre (0, -11.125) radius 3.1
  line L0 (7, 22.25) -> (-7, 22.25)
  line L1 (-7, 22.25) -> (-7, 32.25)
  line L2 (-7, 32.25) -> (7, 32.25)
  line L3 (7, 32.25) -> (7, 22.25)
  line L4 (-7, -22.25) -> (7, -22.25)
  line L5 (7, -22.25) -> (7, -32.25)
  line L6 (7, -32.25) -> (-7, -32.25)
  line L7 (-7, -32.25) -> (-7, -22.25)
  line L8 (30, 89) -> (-30, 89)
  line L9 (-30, 89) -> (-30, -89)
  line L10 (-30, -89) -> (30, -89)
  line L11 (30, -89) -> (30, 89)
  line L12 (15, 37.5) -> (-15, 37.5)
  line L13 (-15, 37.5) -> (-15, -37.5)
  line L14 (-15, -37.5) -> (15, -37.5)
  line L15 (15, -37.5) -> (15, 37.5)
  line L16 (15, 37.5) -> (-15, -37.5) construction
  line L17 (-15, 37.5) -> (15, -37.5) construction
  circle A2 centre (0, 11.125) radius 2.9
  circle A3 centre (0, -11.125) radius 2.9
  dimension "d190" = 75
  dimension "d191" = 30
  dimension "d199" = 5.8
  dimension "d200" = 5.8
  constraint perpendicular L12 L13
  constraint parallel L12 L14
  constraint parallel L13 L15
  constraint horizontal L12
  constraint coincident L16 origin
  constraint coincident L17 origin
  constraint concentric A0 A2
  constraint concentric A1 A3
  measures "d190" distance of L12.end L13.end
  measures "d191" distance of L13.end L14.end
  measures "d199" diameter of A2
  measures "d200" diameter of A3
extrude "Extrude1''''" add sketch "Sketch2 (2)" along normal blind 56 separate body contours A0 | A1 | L0 L1 L2 L3 | L4 L5 L6 L7 | L12 L13 L14 L15 | A2 | A3 makes body 6 in component "ESP Case"
extrude "Extrude2'''" add sketch "Sketch2 (2)" along normal blind 2 contours A0 | A1 | L12 L13 L14 L15 | A2 | A3 bodies 6 in component "ESP Case"
shell "Shell2" thickness 2 removed faces 1 at (-75.6667, 15, 12.5) on bodies 6 in component "ESP Case"
extrude "Extrude4''" add sketch "Sketch2 (2)" against normal blind 1.9 contours A2 | A3 bodies 6 in component "ESP Case"
extrude "Extrude5''" cut sketch "Sketch2 (2)" along normal blind 7 contours L0 L1 L2 L3 | L4 L5 L6 L7 bodies 6 in component "ESP Case"
sketch "Sketch3" plane through (0, -13, 0) normal (0, 1, 0) x (-1, 0, 0) in component "ESP Case"
  line L0 (111, 35.5) -> (59, 35.5)
  line L1 (59, 35.5) -> (59, -35.5)
  line L2 (59, -35.5) -> (111, -35.5)
  line L3 (111, -35.5) -> (111, 35.5)
  line L4 (60, 35) -> (110, 35)
  line L5 (110, 35) -> (110, -35)
  line L6 (110, -35) -> (60, -35)
  line L7 (60, -35) -> (60, 35)
  line L8 (60, 35) -> (110, -35) construction
  line L9 (110, 35) -> (60, -35) construction
  line L10 (110, 32.6888) -> (109.2, 32.6888)
  line L11 (107.68, 35) -> (107.68, 34.2)
  circle A0 centre (107.9239, 32.6803) radius 1.55
  circle A1 centre (62.0226, 32.6803) radius 1.55
  circle A2 centre (62.0226, -33.1306) radius 1.55
  circle A3 centre (107.9239, -33.1306) radius 1.55
  line L12 (107.9239, -33.1306) -> (62.9757, -33.1306)
  line L13 (107.9239, 32.6803) -> (62.0226, 32.6803)
  line L14 (107.9239, -33.1306) -> (107.9239, 32.6803)
  line L15 (62.0226, -33.1306) -> (62.0226, 32.6803)
  line L16 (62.0226, 32.6803) -> (62.0226, -33.1306)
  line L17 (62.9757, -33.1306) -> (62.0226, -33.1306)
  circle A4 centre (107.9239, -33.1306) radius 3.0761
  circle A5 centre (62.0226, -33.1306) radius 3.0226
  circle A6 centre (62.0226, 32.6803) radius 3.0226
  circle A7 centre (107.9239, 32.6803) radius 3.0761
  point P0 (85, 0)
  dimension "d206" = 70
  dimension "d207" = 50
  dimension "d208" = 0.8
  dimension "d209" = 0.8
  dimension "d210" = 3.1
  dimension "d213" = 3.1
  dimension "d214" = 3.1
  dimension "d215" = 3.1
  constraint perpendicular L4 L5
  constraint parallel L4 L6
  constraint parallel L5 L7
  constraint horizontal L4
  constraint coincident L8 P0
  constraint coincident L9 P0
  constraint coincident L5 L10.start
  constraint perpendicular L5 L10
  constraint coincident L4 L11.start
  constraint perpendicular L4 L11
  constraint horizontal L12
  constraint coincident A3.centre L12.start
  constraint horizontal L13
  constraint coincident A0.centre L13.start
  constraint coincident A1.centre L13.end
  constraint vertical L14
  constraint coincident A2.centre L15.start
  constraint vertical L16
  constraint parallel L15 L16
  constraint horizontal L17
  constraint concentric A3 A4
  constraint tangent L3 A4
  constraint concentric A2 A5
  constraint tangent L1 A5
  constraint concentric A1 A6
  constraint tangent L1 A6
  constraint concentric A0 A7
  constraint tangent L3 A7
  measures "d206" distance of L4.end L5.end
  measures "d207" distance of L5.end L6.end
  measures "d208" distance of L10.start L10.end
  measures "d209" distance of L11.start L11.end
  measures "d210" diameter of A0
  measures "d213" diameter of A1
  measures "d214" diameter of A2
  measures "d215" diameter of A3
extrude "Extrude6''" add sketch "Sketch3" along normal blind 15 contours L0 L3 L4 L5 A7 | L0 L4 A7 | L5 A7 | L4 L5 L10 L11 A0 A7 | L2 L5 L6 A4 | L2 L3 A4 | L5 L10 A0 L14 A7 | L0 L4 A6 | L4 L11 A0 L13 A7 | L5 L6 A3 L12 L14 A4 | L2 A4 | A0 L13 L14 A7 | L0 L1 L4 L7 A6 | L4 L7 A1 L13 L15 L16 A6 | A3 L12 L14 A4 | A1 L13 L15 L16 A6 | L2 A5 | L2 L6 L7 A5 | L7 A6 | L6 L7 A2 L12 L15 L16 A5 | A2 L12 L15 L16 A5 | L1 L2 A5 bodies 6 in component "ESP Case"
sketch "Sketch4" plane through (-111, 0, 0) normal (1, 0, 0) x (0, 1, 0) in component "ESP Case"
  line L0 (2, -33.1306) -> (2, -35.5)
  line L1 (2, -35.5) -> (15, -35.5)
  line L2 (15, -35.5) -> (15, 35.5)
  line L3 (15, 35.5) -> (2, 35.5)
  line L4 (2, 35.5) -> (2, 32.6803)
  line L5 (2, 32.6803) -> (-13, 32.6803)
  line L6 (-13, 32.6803) -> (-13, -33.1306)
  line L7 (-13, -33.1306) -> (2, -33.1306)
  line L8 (2, -33.1306) -> (2, 0)
  line L9 (2, 0) -> (12, 0)
  line L10 (2, -27.8732) -> (12, -27.8732)
  line L11 (12, -27.8732) -> (12, -14.8732)
  line L12 (12, -14.8732) -> (2, -14.8732)
  dimension "d218" = 10
  dimension "d219" = 10
  dimension "d220" = 13
  constraint coincident L0.start L7.end
  constraint perpendicular L7 L8
  constraint perpendicular L0 L9
  constraint coincident L8 L10.start
  constraint perpendicular L8 L10
  constraint perpendicular L10 L11
  constraint perpendicular L11 L12
  constraint coincident L8 L12.end
  measures "d218" distance of L8.end L9.end
  measures "d219" distance of L10.start L10.end
  measures "d220" distance of L10.end L11.end
extrude "Extrude7''" cut sketch "Sketch4" against normal blind 22 contours L8 L10 L11 L12 bodies 6 in component "ESP Case"
sketch "Sketch1 (3)" plane through (0, 15, 0) normal (0, 1, 0) x (-1, 0, 0) in component "esp case cover"
  line L0 (59, 35.5) -> (111, 35.5)
  line L1 (111, 35.5) -> (111, -35.5)
  line L2 (111, -35.5) -> (59, -35.5)
  line L3 (59, -35.5) -> (59, 35.5)
  line L4 (57, -37.5) -> (113, -37.5)
  line L5 (113, -37.5) -> (113, 37.5)
  line L6 (113, 37.5) -> (57, 37.5)
  line L7 (57, 37.5) -> (57, -37.5)
  line L8 (57, 37.5) -> (113, 37.5)
  line L9 (113, 37.5) -> (113, -37.5)
  line L10 (113, -37.5) -> (57, -37.5)
  line L11 (57, -37.5) -> (57, 37.5)
  line L12 (111, -35.5) -> (59, -35.5)
  line L13 (59, -35.5) -> (59, 35.5)
  line L14 (59, 35.5) -> (111, 35.5)
  line L15 (111, 35.5) -> (111, -35.5)
  line L16 (59, 35.5) -> (60.4142, 34.0858)
  line L17 (59, 35.5) -> (61, 35.5) construction
  line L18 (111, 35.5) -> (109.5858, 34.0858)
  line L19 (111, 35.5) -> (109, 35.5) construction
  line L20 (111, -35.5) -> (109.5858, -34.0858)
  line L21 (111, -35.5) -> (109, -35.5) construction
  line L22 (59, -35.5) -> (60.4142, -34.0858)
  line L23 (59, -35.5) -> (61, -35.5) construction
  line L24 (60.4142, 34.0858) -> (109.5858, 34.0858)
  line L25 (109.5858, 34.0858) -> (109.5858, -34.0858)
  line L26 (109.5858, -34.0858) -> (60.4142, -34.0858)
  line L27 (60.4142, -34.0858) -> (60.4142, 34.0858)
  dimension "d223" = 45
  dimension "d224" = 2
  dimension "d225" = 45
  dimension "d226" = 2
  dimension "d227" = 45
  dimension "d228" = 2
  dimension "d229" = 45
  dimension "d230" = 2
  constraint horizontal L8
  constraint vertical L9
  constraint horizontal L10
  constraint vertical L11
  constraint coincident L4.end L5.start
  constraint coincident L6.end L7.start
  constraint horizontal L12
  constraint vertical L13
  constraint horizontal L14
  constraint vertical L15
  constraint coincident L0.start L3.end
  constraint coincident L1.end L2.start
  constraint horizontal L17
  constraint horizontal L19
  constraint horizontal L21
  constraint horizontal L23
  constraint horizontal L24
  constraint vertical L25
  constraint horizontal L26
  constraint vertical L27
  measures "d223" angle of L16 L17
  measures "d224" distance of L0.start L16.end
  measures "d225" angle of L18 L19
  measures "d226" distance of L0.end L18.end
  measures "d227" angle of L20 L21
  measures "d228" distance of L1.end L20.end
  measures "d229" angle of L22 L23
  measures "d230" distance of L2.end L22.end
extrude "Extrude1'''''" add sketch "Sketch1 (3)" along normal blind 2 separate body contours L3 L13 L16 L22 L27 | L0 L14 L16 L18 L24 | L1 L15 L18 L20 L25 | L2 L12 L20 L22 L26 | L24 L25 L26 L27 | L4 L5 L6 L7 L8 L9 L10 L11 makes body 7 in component "esp case cover"
extrude "Extrude2''''" add sketch "Sketch1 (3)" against normal blind 3 contours L3 L13 L16 L22 L27 | L0 L14 L16 L18 L24 | L1 L15 L18 L20 L25 | L2 L12 L20 L22 L26 bodies 7 in component "esp case cover"
extrude "Extrude8''" add 1 faces at (-113, 0.6667, 20.0423) along direction (-1, 0, 0) blind 10 on bodies 6 bodies 6 in component "ESP Case"
ref_plane "WorkPlane1" through (-90, 0, 0) normal (0, 1, 0) x (0, 0, -1) in component "ESP Case"
sketch "haken ffnung" plane through (-90, 0, 0) normal (0, 1, 0) x (1, 0, 0) in component "ESP Case"
  line L0 (-33, -19) -> (-30, -19)
  line L1 (-28.5, -20.5) -> (-28.5, -28)
  line L2 (-28.5, -28) -> (-25.4, -28)
  line L3 (-25.4, -28) -> (-25.4, -5)
  line L4 (-25.4, -5) -> (-33, -5)
  line L5 (-33, -5) -> (-33, -19)
  arc A0 (-28.5, -20.5) -> (-30, -19) centre (-30, -20.5) ccw
  point P0 (-28.5, -19)
  dimension "d238" = 4.5
  dimension "d239" = 3.1
  dimension "d243" = 14
  dimension "d244" = 9
  dimension "d247" = 1.5
  constraint horizontal L0
  constraint perpendicular L0 L1
  constraint perpendicular L1 L2
  constraint perpendicular L2 L3
  constraint perpendicular L3 L4
  constraint perpendicular L0 L5
  constraint coincident P0 L0
  constraint coincident P0 L1
  constraint tangent L0 A0
  constraint tangent L1 A0
  measures "d238" distance of L0.start P0
  measures "d239" distance of L1.end L2.end
  measures "d243" distance of L0.start L4.end
  measures "d244" distance of P0 L1.end
  measures "d247" radius of A0
extrude "Extrude9'" cut sketch "haken ffnung" along normal mid plane 6.28 bodies 6 in component "ESP Case"
extrude "Extrude3'''" add 1 faces at (-113, 15.6667, -12.5) along direction (-1, 0, 0) blind 10 on bodies 7 bodies 7 in component "esp case cover"
component "led divider" placed x (1, 0, 0) y (0, 1, 0) z (0, 0, 1) at (0, 0, 0)
component "LED plate" placed x (1, 0, 0) y (0, 1, 0) z (0, 0, 1) at (0, 0, 0)
component "glass" placed x (1, 0, 0) y (0, 1, 0) z (0, 0, 1) at (0, 27, 0)
component "case" placed x (1, 0, 0) y (0, 1, 0) z (0, 0, 1) at (0, 0, 0)
component "ESP Case" placed x (1, 0, 0) y (0, 1, 0) z (0, 0, 1) at (0, 0, 0)
component "esp case cover" placed x (1, 0, 0) y (0, 1, 0) z (0, 0, 1) at (0, 0, 0) in component "ESP Case"
equation "d66 = ( 60 / 2 ) * 1 mm"
equation "d68 = ( 60 / 2 ) * 1 mm - 3.2 mm"
equation "d70 = ( 60 / 2 ) * 1 mm - 4.2 mm"
